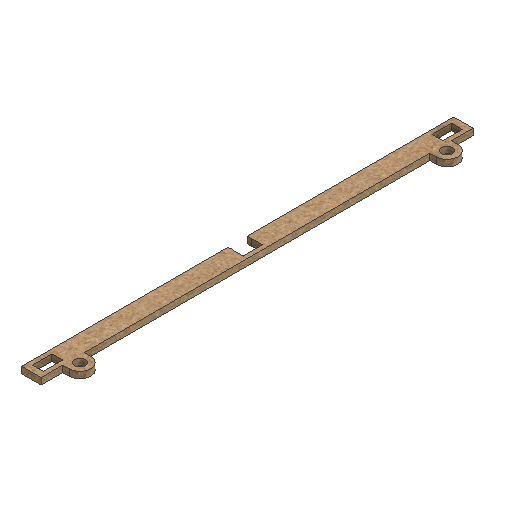
# Autodesk Inventor part: Lower_Bar
Saved by Autodesk Inventor 2024 (Build 280153000, 153)
## iProperties
Created: 2024-04-09
Part Number: Lower_Bar
Material: MDF Medium Density Fiberboard
Document SubType Name: Modeling
Designer: USER
Density: 0.8 g/cm^3
Appearance: Cardboard - Corrugated
Mass: 4.19201 g
Surface Area: 51.2327 cm^2
Volume: 5.24001 cm^3
Author: USER
Autodesk Inventor part; units mm, degrees
ref_plane "YZ Plane" through (0, 0, 0) normal (1, 0, 0) x (0, 1, 0)
ref_plane "XZ Plane" through (0, 0, 0) normal (0, 1, 0) x (-1, 0, 0)
ref_plane "XY Plane" through (0, 0, 0) normal (0, 0, 1) x (1, 0, 0)
sketch "草圖1" plane through (0, 0, 0) normal (0, 1, 0) x (-1, 0, 0)
  line L0 (0, 80) -> (9, 80)
  line L1 (9, -80) -> (0, -80)
  line L2 (0, -80) -> (0, 80)
  line L3 (7, 4.5) -> (2, 4.5)
  line L4 (2, 4.5) -> (2, -4.5)
  line L5 (2, -4.5) -> (7, -4.5)
  line L6 (9, 80) -> (9, 90)
  line L7 (9, 90) -> (-3, 90)
  line L8 (-8, 85) -> (-8, 85)
  line L9 (-3, 80) -> (0, 80)
  arc A0 (-8, 85) -> (-3, 80) centre (-3, 85) ccw
  arc A1 (-3, 90) -> (-8, 85) centre (-3, 85) ccw
  circle A2 centre (-3, 85) radius 2.5
  line L10 (9, 0) -> (0, 0)
  line L11 (9, -80) -> (9, -90)
  line L12 (9, -90) -> (-3, -90)
  line L13 (-3, -80) -> (0, -80)
  arc A3 (-3, -80) -> (-8, -85) centre (-3, -85) ccw
  arc A4 (-8, -85) -> (-3, -90) centre (-3, -85) ccw
  circle A5 centre (-3, -85) radius 2.5
  line L14 (9, 80) -> (9, 4.6)
  line L15 (9, -4.6) -> (9, -80)
  line L16 (7, -4.5) -> (7, -4.2)
  line L17 (7, -4.2) -> (9, -4.6)
  line L18 (7, 4.5) -> (7, 4.2)
  line L19 (7, 4.2) -> (9, 4.6)
  line L20 (9, 90) -> (0, 90)
  line L21 (0, 90) -> (0, 100)
  line L22 (0, 100) -> (9, 100)
  line L23 (9, 100) -> (9, 90)
  line L24 (9, -90) -> (0, -90)
  line L25 (0, -90) -> (0, -100)
  line L26 (0, -100) -> (9, -100)
  line L27 (9, -100) -> (9, -90)
  line L28 (2, 97) -> (7, 97)
  line L29 (7, 97) -> (7, 88)
  line L30 (7, 88) -> (2, 88)
  line L31 (2, 88) -> (2, 97)
  line L32 (7, -97) -> (2, -97)
  line L33 (2, -97) -> (2, -88)
  line L34 (2, -88) -> (7, -88)
  line L35 (7, -88) -> (7, -97)
  point P0 (4.5, 4.5)
  point P1 (4.5, 80)
  point P2 (-8, 90)
  point P3 (-8, -90)
  point P4 (2, 0)
  point P5 (4.5, 97)
  point P6 (4.5, 100)
  point P7 (4.5, -97)
  point P8 (4.5, -100)
  dimension "d0" = 160
  dimension "d1" = 9
  dimension "d3" = 5
  dimension "d4" = 10
  dimension "d5" = 17
  dimension "d6" = 5
  dimension "d7" = 5
  dimension "d8" = 5
  dimension "d13" = 9
  dimension "d14" = 0.3
  dimension "d15" = 0.3
  dimension "d17" = 0
  dimension "d18" = 5
  dimension "d21" = 17
  dimension "d22" = 10
  dimension "d23" = 9
  dimension "d24" = 9
  dimension "d25" = 10
  dimension "d26" = 9
  dimension "d27" = 5
  dimension "d28" = 3
  dimension "d29" = 9
  dimension "d30" = 5
  dimension "d31" = 3
  dimension "d32" = 75.4
  dimension "d33" = 75.4
  constraints: 72 end point, 13 parallel, 10 perpendicular, 9 symmetric about line, 8 midpoint, 8 point on circle, 7 horizontal, 6 centre point, 4 tangent, 3 coincident, 3 point on line, 3 vertical, 3 vertical alignment, 1 horizontal alignment, 3 other
  measures "d0" distance of L0.end L1.start
  measures "d1" distance of L0.start L0.end
  measures "d3" distance of L4.end L5.end
  measures "d4" distance of L0.end L6.end
  measures "d5" distance of L6.end point (-8, 90)
  measures "d6" radius of A0
  measures "d7" radius of A1
  measures "d8" diameter of A2
  measures "d13" distance of L3.end L4.end
  measures "d14" distance of L5.end L16.end
  measures "d15" distance of L3.start L18.end
  measures "d17" distance from line of L10.start L15
  measures "d18" distance from line of point (-8, 85) L0
  measures "d21" distance from line of point (-8, -85) L15
  measures "d22" distance of L22.end L6.end
  measures "d23" distance of L21.end L22.end
  measures "d24" distance of L25.end L26.end
  measures "d25" distance of L26.end L12.start
  measures "d26" distance of L28.end L29.end
  measures "d27" distance of L29.end L30.end
  measures "d28" vertical distance of L21.end L28.start
  measures "d29" distance of L32.end L33.end
  measures "d30" distance of L33.end L34.end
  measures "d31" distance between parallel lines of L26 L32
  measures "d32" distance of L0.end L14.end
  measures "d33" distance of L15.start L1.start
extrude "擠出1" add sketch "草圖1" along normal blind 3 contours L9 A0 A1 L7 L31 L30 L29 L6 L0 | L0 L14 L19 L18 L3 L4 L10 L2 | L10 L4 L5 L16 L17 L15 L1 L2 | L7 L29 L28 L31 L21 L22 L23 | L1 L11 L12 L35 L34 L33 A4 A3 L13 | L27 L26 L25 L12 L33 L32 L35
